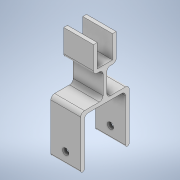
# Autodesk Inventor part: back_wheel_interface
Saved by Autodesk Inventor 2021 (Build 250183000, 183)
## iProperties
Created: 2020-12-01
Part Number: back_wheel_interface
Material: Generic
Document SubType Name: Modeling
Designer: Semester Project
Density: 1 g/cm^3
Appearance: Default
Mass: 0.511577 g
Surface Area: 11.3423 cm^2
Volume: 0.511577 cm^3
Author: Semester Project
Autodesk Inventor part; units mm, degrees
ref_plane "YZ Plane" through (0, 0, 0) normal (1, 0, 0) x (0, 1, 0)
ref_plane "XZ Plane" through (0, 0, 0) normal (0, 1, 0) x (-1, 0, 0)
ref_plane "XY Plane" through (0, 0, 0) normal (0, 0, 1) x (1, 0, 0)
sketch "Sketch1" plane through (0, 0, 0) normal (1, 0, 0) x (0, 1, 0)
  line L0 (-232.9787, 228.8989) -> (-240.0787, 228.8989)
  line L1 (-240.0787, 228.8989) -> (-240.0787, 226.3489)
  line L2 (-240.0787, 226.3489) -> (-247.0787, 226.3489)
  line L3 (-261.0787, 231.3489) -> (-248.0787, 231.3489)
  line L4 (-232.9787, 228.8989) -> (-232.9787, 227.8989)
  line L5 (-232.9787, 227.8989) -> (-239.0787, 227.8989)
  line L6 (-239.0787, 227.8989) -> (-239.0787, 227.8489)
  line L7 (-258.789, 225.8489) -> (279.9992, 225.8489) construction
  line L8 (-232.9787, 222.7989) -> (-240.0787, 222.7989)
  line L9 (-240.0787, 222.7989) -> (-240.0787, 225.3489)
  line L10 (-240.0787, 225.3489) -> (-247.0787, 225.3489)
  line L11 (-261.0787, 220.3489) -> (-248.0787, 220.3489)
  line L12 (-232.9787, 222.7989) -> (-232.9787, 223.7989)
  line L13 (-232.9787, 223.7989) -> (-239.0787, 223.7989)
  line L14 (-239.0787, 223.7989) -> (-239.0787, 227.8489)
  line L15 (-248.0787, 231.3489) -> (-248.0787, 220.3489)
  line L16 (-261.0787, 231.3489) -> (-261.0787, 232.3489)
  line L17 (-261.0787, 232.3489) -> (-247.0787, 232.3489)
  line L18 (-247.0787, 232.3489) -> (-247.0787, 226.3489)
  line L19 (-247.0787, 225.3489) -> (-247.0787, 219.3489)
  line L20 (-247.0787, 219.3489) -> (-261.0787, 219.3489)
  line L21 (-261.0787, 219.3489) -> (-261.0787, 220.3489)
  point P0 (0, 0)
  dimension "d4" = 1
  dimension "d6" = 4.1
  dimension "d9" = 1
  dimension "d10" = 1
  dimension "d13" = 6.1
  dimension "d14" = 11
  dimension "d15" = 1
  dimension "d16" = 1
  dimension "d17" = 1
  dimension "d29" = 13
  dimension "d32" = 7
  constraints: 44 end point, 8 symmetric about line, 7 perpendicular, 2 horizontal, 2 parallel, 2 point on line, 2 vertical
  measures "d4" distance between parallel lines of L10 L2
  measures "d6" distance between parallel lines of L13 L5
  measures "d9" distance between parallel lines of L9 L14
  measures "d10" distance between parallel lines of L5 L0
  measures "d13" distance of L4.end L5.end
  measures "d14" distance of L3.end L11.end
  measures "d15" distance of L20.end L11.start
  measures "d16" distance of L3.start L16.end
  measures "d17" distance between parallel lines of L18 L15
  measures "d29" distance of L11.start L11.end
  measures "d32" distance of L1.end L2.end
extrude "Extrusion1" add sketch "Sketch1" along normal blind 8
sketch "Sketch2" plane through (0, -261.0787, 219.3489) normal (0, 0, -1) x (-1, 0, 0)
  line L0 (0, 14) -> (-8, 14) projected
  line L1 (0, 0) -> (0, 14) projected
  point P0 (0, 261.0787)
  point P1 (-4, 3)
  dimension "d25" = 11
  dimension "d26" = 4
  dimension "d27" = 8
  dimension "d28" = 14
  measures "d25" distance from line of L0 point (-4, 3)
  measures "d26" distance from line of L1 point (-4, 3)
  measures "d27" distance of L0.start L0.end
  measures "d28" distance of L1.start L0.start
hole "Hole1" at (4, -258.0787, 219.3489) direction (0, 0, 1) diameter 1.7 end through all
fillet "Fillet1" radius 0.5 4 edges at (4, -261.0787, 231.3489) (4, -261.0787, 232.3489) (4, -261.0787, 220.3489) (4, -261.0787, 219.3489)
fillet "Fillet2" radius 1 10 edges at (4, -247.0787, 232.3489) (4, -248.0787, 231.3489) (4, -247.0787, 219.3489) (4, -248.0787, 220.3489) (4, -247.0787, 225.3489) (4, -247.0787, 226.3489) (4, -240.0787, 226.3489) (4, -240.0787, 222.7989) (4, -240.0787, 225.3489) (4, -240.0787, 228.8989)
equation "\"d26\" = 0.5 * d27"
body "Solid1"
